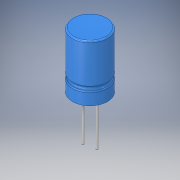
# Autodesk Inventor part: CAP12.5X20
Saved by Autodesk Inventor 2018 (Build 220112000, 112)
## iProperties
Created: 2018-02-21
Part Number: CAP12.5X20
Material: PC/ABS Plastic
Document SubType Name: Modeling
Designer: brutu
Density: 0.357273 g/cm^3
Appearance: Cyan
Author: brutu
Autodesk Inventor part; units mm, degrees
ref_plane "YZ Plane" through (0, 0, 0) normal (1, 0, 0) x (0, 1, 0)
ref_plane "XZ Plane" through (0, 0, 0) normal (0, 1, 0) x (-1, 0, 0)
ref_plane "XY Plane" through (0, 0, 0) normal (0, 0, 1) x (1, 0, 0)
sketch "Sketch1" plane through (0, 0, 0) normal (0, 0, 1) x (1, 0, 0)
  line L0 (0, 5.3298) -> (6.25, 5.3298)
  line L1 (6.25, -14.6702) -> (0, -14.6702)
  line L2 (0, -14.6702) -> (0, 5.3298)
  circle A0 centre (6.25, -9.5902) radius 0.635
  line L3 (6.25, 5.3298) -> (6.25, -8.9552)
  line L4 (6.25, -10.2252) -> (6.25, -14.6702)
  point P0 (0, 0)
  dimension "d0" = 6.25
  dimension "d1" = 20
  dimension "d2" = 1.27
  dimension "d3" = 5.08
  constraints: 10 end point, 2 point on circle, 1 centre point, 1 collinear, 1 horizontal, 1 parallel, 1 point on line, 1 vertical
  measures "d0" distance of L0.start L0.end
  measures "d1" distance of L0.end L1.start
  measures "d2" diameter of A0
  measures "d3" distance from line of L1 A0.centre
revolve "Revolution1" add sketch "Sketch1" angle 360 about axis through (0, -14.6702, 0) along (0, 1, 0) contours L0 L3 A0 L4 L1 L2
fillet "Fillet1" radius 0.508 3 edges at (-6.25, -10.2252, 0) (-6.25, -8.9552, 0) (-6.25, 5.3298, 0)
sketch "Sketch2" plane through (0, -14.6702, 0) normal (0, -1, 0) x (1, 0, 0)
  circle A0 centre (0, 2.5) radius 0.3
  circle A1 centre (0, -2.5) radius 0.3
  point P0 (0, 0)
  dimension "d6" = 0.6
  dimension "d7" = 0.6
  dimension "d8" = 2.5
  dimension "d9" = 2.5
  constraints: 2 centre point
  measures "d6" diameter of A0
  measures "d7" diameter of A1
  measures "d8" distance of A0.centre point (0, 0)
  measures "d9" distance of A1.centre point (0, 0)
extrude "Extrusion1" add sketch "Sketch2" along normal blind 15
sketch "Sketch3" plane through (0, -29.6702, -2.5) normal (0, -1, 0) x (1, 0, 0)
  circle A0 centre (0, 0) radius 0.3 projected
  point P0 (0, 2.5)
extrude "Extrusion2" add sketch "Sketch3" along normal blind 4
equation "\"d7\" = d6"
body "Solid1"
